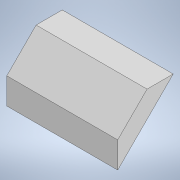
# Autodesk Inventor part: shelf
Saved by Autodesk Inventor 2020 (Build 240168000, 168)
## iProperties
Created: 2021-11-03
Part Number: shelf
Material: Generic
Document SubType Name: Modeling
Designer: 17185
Density: 1 g/cm^3
Appearance: Default
Author: 17185
Autodesk Inventor part; units mm, degrees
ref_plane "YZ Plane" through (0, 0, 0) normal (1, 0, 0) x (0, 1, 0)
ref_plane "XZ Plane" through (0, 0, 0) normal (0, 1, 0) x (-1, 0, 0)
ref_plane "XY Plane" through (0, 0, 0) normal (0, 0, 1) x (1, 0, 0)
sketch "Sketch1" plane through (0, 0, 0) normal (1, 0, 0) x (0, 1, 0)
  line L0 (19.05, 19.05) -> (-19.05, 19.05) construction
  line L1 (-19.05, 19.05) -> (-19.05, -19.05) construction
  line L2 (-19.05, -19.05) -> (19.05, -19.05) construction
  line L3 (19.05, -19.05) -> (19.05, 19.05) construction
  line L4 (19.05, 19.05) -> (-19.05, -19.05) construction
  line L5 (-19.05, 19.05) -> (19.05, -19.05) construction
  line L6 (-19.05, 19.05) -> (19.05, -19.05)
  line L7 (19.05, -1.0895) -> (-1.0895, 19.05)
  line L8 (-19.05, 19.05) -> (-1.0895, 19.05)
  line L9 (19.05, -1.0895) -> (19.05, -19.05)
  point P0 (0, 0)
  dimension "d0" = 38.1
  dimension "d1" = 38.1
  dimension "d2" = 12.7
  constraints: 20 end point, 3 parallel, 2 midpoint, 2 point on line, 1 horizontal, 1 perpendicular, 1 vertical
  measures "d0" distance of L1.end L2.end
  measures "d1" distance of L0.end L1.end
  measures "d2" distance between parallel lines of L5 L7
extrude "Extrusion1" add sketch "Sketch1" along normal blind 76.2
body "Solid1"
